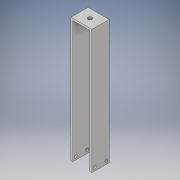
# Autodesk Inventor part: Part11
Saved by Autodesk Inventor 2019.1 (Build 231200000, 200)
## iProperties
Created: 2018-09-18
Part Number: Part11
Material: Generic
Document SubType Name: Modeling
Designer: drawing
Density: 1 g/cm^3
Appearance: Default
Author: drawing
Autodesk Inventor part; units mm, degrees
ref_plane "YZ Plane" through (0, 0, 0) normal (1, 0, 0) x (0, 1, 0)
ref_plane "XZ Plane" through (0, 0, 0) normal (0, 1, 0) x (-1, 0, 0)
ref_plane "XY Plane" through (0, 0, 0) normal (0, 0, 1) x (1, 0, 0)
sketch "Sketch1" plane through (0, 0, 0) normal (0, 0, 1) x (1, 0, 0)
  line L0 (0, 0) -> (28.575, 0)
  line L1 (28.575, 0) -> (28.575, 203.2)
  line L2 (28.575, 203.2) -> (0, 203.2)
  line L3 (0, 203.2) -> (0, 0)
  line L4 (31.75, 206.375) -> (31.75, 0)
  line L5 (-3.175, 0) -> (-3.175, 206.375)
  line L6 (-3.175, 206.375) -> (31.75, 206.375)
  line L7 (-3.175, 0) -> (31.75, 0)
  dimension "d0" = 28.575
  dimension "d1" = 203.2
  dimension "d2" = 3.175
  dimension "d24" = 3.175
  dimension "d25" = 3.175
  constraints: 16 end point, 3 parallel, 1 horizontal, 1 perpendicular, 1 point on line
  measures "d0" distance of L2.end L1.end
  measures "d1" distance of L1.end L0.end
  measures "d2" distance between parallel lines of L1 L4
  measures "d24" distance between parallel lines of L2 L6
  measures "d25" distance between parallel lines of L3 L5
extrude "Extrusion1" add sketch "Sketch1" along normal blind 28.575 contours L7 L5 L6 L4 L1 L2 L3
sketch "Sketch2" plane through (31.75, 0, 0) normal (1, 0, 0) x (0, 0, -1)
  line L0 (0, 0) -> (-28.575, 0) projected
  line L1 (0, 206.375) -> (0, 0) projected
  point P0 (-23.8125, 5.207)
  point P1 (-4.7625, 5.207)
  dimension "d5" = 5.207
  dimension "d6" = 19.05
  dimension "d7" = 28.575
  dimension "d8" = 4.7625
  constraints: 1 horizontal alignment
  measures "d5" distance from line of point (-4.762, 5.207) L0
  measures "d6" distance of point (-23.812, 5.207) point (-4.762, 5.207)
  measures "d7" distance of L0.start L0.end
  measures "d8" distance from line of L1 point (-4.762, 5.207)
hole "Hole1" at (31.75, 5.207, 23.8125) at (31.75, 5.207, 4.7625) direction (-1, 0, 0) diameter 5.1054 end through all clearance for "Flat Head Machine Screw (82)" size "#10" standard "Ansi Unified Screw Threads"
sketch "Sketch3" plane through (-3.175, 206.375, 0) normal (0, 1, 0) x (1, 0, 0)
  line L0 (3.175, 0) -> (3.175, -28.575) projected
  line L1 (31.75, 0) -> (31.75, -28.575) projected
  point P0 (17.4625, -14.2875)
  point P1 (3.175, -14.2875)
  dimension "d16" = 14.2875
  constraints: 1 horizontal alignment, 1 midpoint
  measures "d16" distance from line of L0 point (17.463, -14.287)
hole "Hole2" at (14.2875, 206.375, 14.2875) direction (0, -1, 0) diameter 6.7564 end through all clearance for "Flat Head Machine Screw (82)" size "1/4" standard "Ansi Unified Screw Threads"
equation "\"d8\" = -0.5 * d6 + 0.5 * d7"
body "Solid1"
